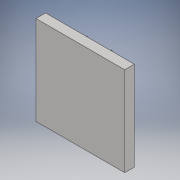
# Autodesk Inventor part: Logo
Saved by Autodesk Inventor 2018 (Build 220112000, 112)
## iProperties
Created: 2019-02-22
Part Number: Logo
Material: Generic
Document SubType Name: Modeling
Designer: This kid
Density: 1 g/cm^3
Appearance: Default
Author: This kid
Autodesk Inventor part; units mm, degrees
ref_plane "YZ Plane" through (0, 0, 0) normal (1, 0, 0) x (0, 1, 0)
ref_plane "XZ Plane" through (0, 0, 0) normal (0, 1, 0) x (-1, 0, 0)
ref_plane "XY Plane" through (0, 0, 0) normal (0, 0, 1) x (1, 0, 0)
sketch "Sketch4" plane through (0, 0, 0) normal (0, 0, 1) x (1, 0, 0)
  line L0 (-28.9374, -10.0235) -> (-36.7376, -0.0011)
  line L1 (-28.9374, -10.0235) -> (-16.2374, -10.0235) construction
  line L2 (-36.7376, -0.0011) -> (-15.7934, 29.7213)
  line L3 (-15.7934, 29.7213) -> (-28.9374, -10.0235)
  line L4 (0, 0) -> (0, 43.134) construction
  line L5 (0, -17.5109) -> (-45.4613, -17.5109) construction
  line L6 (-45.4613, -17.5109) -> (54.0034, -17.5109) construction
  line L7 (28.9374, -10.0235) -> (36.7376, -0.0011)
  line L8 (36.7376, -0.0011) -> (15.7934, 29.7213)
  line L9 (15.7934, 29.7213) -> (28.9374, -10.0235)
  line L10 (-28.9374, -24.9984) -> (-36.7376, -35.0207)
  line L11 (-36.7376, -35.0207) -> (-15.7934, -64.7432)
  line L12 (-15.7934, -64.7432) -> (-28.9374, -24.9984)
  line L13 (15.7934, -64.7432) -> (28.9374, -24.9984)
  line L14 (36.7376, -35.0207) -> (15.7934, -64.7432)
  line L15 (28.9374, -24.9984) -> (36.7376, -35.0207)
  dimension "d9" = 12.7
  constraints: 32 end point, 9 symmetric about line, 2 horizontal, 1 equal length, 1 point on line, 1 vertical
  measures "d9" distance of L0.start L0.end
sketch "Sketch5" plane through (0, 0, 0) normal (0, 0, 1) x (1, 0, 0)
  line L0 (-58.3358, 40.999) -> (58.3358, 40.999)
  line L1 (58.3358, 40.999) -> (58.3358, -76.1205)
  line L2 (58.3358, -76.1205) -> (-58.3358, -76.1205)
  line L3 (-58.3358, -76.1205) -> (-58.3358, 40.999)
  line L4 (-58.3358, 40.999) -> (58.3358, -76.1205) construction
  line L5 (58.3358, 40.999) -> (-58.3358, -76.1205) construction
  point P0 (0, 0)
  point P1 (0, -17.5607)
  constraints: 12 end point, 2 midpoint, 2 parallel, 1 horizontal, 1 perpendicular
extrude "Extrusion4" add sketch "Sketch4" against normal blind 25.4
extrude "Extrusion5" add sketch "Sketch5" against normal blind 12.7
sketch "Sketch6" plane through (0, 0, -12.7) normal (0, 0, -1) x (-1, 0, 0)
  line L0 (-23.8244, -6.5433) -> (-21.2379, -6.5433)
  line L1 (-20.9936, 4.8166) -> (-6.9933, 4.8166)
  line L2 (-6.9933, 4.8166) -> (0, -43.0842)
  line L3 (0, -43.0842) -> (8.4371, 5.9599)
  line L4 (8.4371, 5.9599) -> (21.8678, 5.9599)
  line L5 (21.8678, 5.9599) -> (0, -59.2796)
  line L6 (0, -59.2796) -> (-20.9936, 4.8166)
  point P0 (0, 0)
  constraints: 14 end point, 2 horizontal
extrude "Extrusion6" add sketch "Sketch6" along normal blind 12.7
sketch "Sketch7" plane through (0, 0, -12.7) normal (0, 0, -1) x (-1, 0, 0)
  line L0 (-19.319, 35.5552) -> (28.0582, 35.5552) construction
  line L1 (28.0582, 35.5552) -> (28.0582, 31.6649) construction
  line L2 (28.0582, 31.6649) -> (-19.319, 31.6649) construction
  line L3 (-19.319, 31.6649) -> (-19.319, 35.5552) construction
  point P0 (0, 0)
  constraints: 2 other
body "Solid2"
